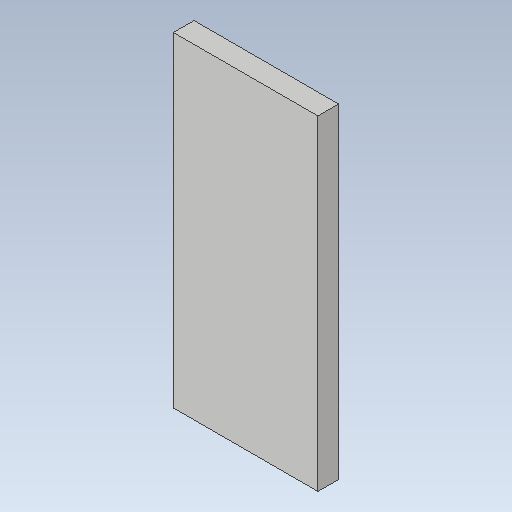
# Autodesk Inventor part: Cross Support 2
Saved by Autodesk Inventor 2021 (Build 250183000, 183)
## iProperties
Created: 2020-12-28
Part Number: Cross Support 2
Material: Generic
Document SubType Name: Modeling
Designer: Thomas Dodd
Density: 1 g/cm^3
Appearance: Default
Author: Thomas Dodd
Autodesk Inventor part; units mm, degrees
ref_plane "YZ Plane" through (0, 0, 0) normal (1, 0, 0) x (0, 1, 0)
ref_plane "XZ Plane" through (0, 0, 0) normal (0, 1, 0) x (-1, 0, 0)
ref_plane "XY Plane" through (0, 0, 0) normal (0, 0, 1) x (1, 0, 0)
sketch "Sketch1" plane through (0, 0, 0) normal (0, 1, 0) x (-1, 0, 0)
  line L0 (0, 0) -> (140, 0)
  line L1 (140, 0) -> (140, -20)
  line L2 (140, -20) -> (0, -20)
  line L3 (0, -20) -> (0, 0)
  dimension "d0" = 140
  dimension "d1" = 20
  constraints: 8 end point, 2 parallel, 1 horizontal, 1 perpendicular
  measures "d0" distance of L1.end L2.end
  measures "d1" distance of L0.end L1.end
extrude "Extrusion1" add sketch "Sketch1" along normal blind 315
sketch "Sketch2" plane through (-140, 0, 0) normal (0, 0, 1) x (1, 0, 0)
  line L0 (140, 0) -> (0, 0) projected
  line L1 (140, 0) -> (140, 315) projected
  line L2 (0, 315) -> (140, 315) projected
  line L3 (0, 0) -> (0, 315) projected
body "Solid1"
